Autodesk Fusion 360 part; units mm, degrees
(part 2 of 4)
  spline S0 degree 5 poles (47.3702, 73.019) (47.3923, 73.0171) (47.4364, 73.0131) (47.5026, 73.0067) (47.5909, 72.9976) (47.701, 72.9852) (47.8111, 72.9719) (47.9211, 72.9579) (48.0309, 72.9431) (48.1407, 72.9277) (48.2504, 72.9116) (48.3599, 72.8948) (48.4693, 72.8773) (48.5786, 72.8591) (48.6878, 72.8403) (48.7969, 72.821) (48.9059, 72.8012) (49.0149, 72.7809) (49.1238, 72.7601) (49.2325, 72.7384) (49.341, 72.7156) (49.4491, 72.6914) (49.5568, 72.6656) (49.6641, 72.6381) (49.771, 72.6091) (49.8776, 72.579) (49.984, 72.5482) (50.0903, 72.517) (50.1965, 72.4856) (50.3027, 72.4541) (50.4087, 72.4222) (50.5146, 72.3898) (50.6202, 72.3565) (50.7255, 72.322) (50.8304, 72.2863) (50.9348, 72.2494) (51.0388, 72.2111) (51.1423, 72.1717) (51.2453, 72.1314) (51.3481, 72.0902) (51.4506, 72.0484) (51.5529, 72.0061) (51.6551, 71.9634) (51.7572, 71.9202) (51.859, 71.8765) (51.9604, 71.8319) (52.0614, 71.7862) (52.1617, 71.7392) (52.2614, 71.6908) (52.3603, 71.6411) (52.4587, 71.5903) (52.5566, 71.5385) (52.6542, 71.486) (52.7515, 71.433) (52.8486, 71.3796) (52.9454, 71.3257) (53.0418, 71.2712) (53.1379, 71.2161) (53.2336, 71.1602) (53.3288, 71.1036) (53.4236, 71.0462) (53.5179, 70.9881) (53.6118, 70.9293) (53.7052, 70.8698) (53.7983, 70.8096) (53.8909, 70.7488) (53.983, 70.6873) (54.0746, 70.625) (54.1658, 70.562) (54.2565, 70.4984) (54.3468, 70.4342) (54.4367, 70.3694) (54.5263, 70.3041) (54.6154, 70.2382) (54.704, 70.1716) (54.792, 70.1041) (54.8791, 70.0356) (54.9653, 69.9659) (55.0505, 69.8951) (55.1349, 69.8232) (55.2187, 69.7506) (55.302, 69.6773) (55.3849, 69.6038) (55.4677, 69.53) (55.5503, 69.456) (55.6325, 69.3816) (55.7141, 69.3067) (55.7951, 69.2309) (55.8751, 69.1542) (55.9542, 69.0764) (56.0322, 68.9977) (56.1093, 68.9179) (56.1854, 68.8373) (56.2607, 68.7559) (56.3353, 68.6739) (56.4094, 68.5914) (56.483, 68.5085) (56.5562, 68.4253) (56.6292, 68.3418) (56.7017, 68.2579) (56.7736, 68.1735) (56.8448, 68.0886) (56.9151, 68.0029) (56.9845, 67.9165) (57.053, 67.8293) (57.1207, 67.7416) (57.1877, 67.6533) (57.2542, 67.5646) (57.3203, 67.4756) (57.3859, 67.3862) (57.4509, 67.2965) (57.5153, 67.2063) (57.5788, 67.1155) (57.6414, 67.0241) (57.703, 66.932) (57.7635, 66.8393) (57.8231, 66.7458) (57.8817, 66.6518) (57.9395, 66.5572) (57.9967, 66.4623) (58.0535, 66.3671) (58.11, 66.2718) (58.1661, 66.1765) (58.2219, 66.0809) (58.2771, 65.985) (58.3312, 65.8884) (58.384, 65.791) (58.4353, 65.6925) (58.4851, 65.5931) (58.534, 65.4932) (58.5826, 65.3934) (58.6315, 65.2941) (58.681, 65.1955) (58.7306, 65.0975) (58.7792, 64.9989) (58.8253, 64.8988) (58.8676, 64.796) (58.9055, 64.69) (58.9398, 64.5816) (58.9733, 64.4726) (59.0098, 64.366) (59.0533, 64.2649) (59.1074, 64.1722) (59.1741, 64.0899) (59.2531, 64.0181) (59.3425, 63.956) (59.4393, 63.9018) (59.5404, 63.8534) (59.6431, 63.8089) (59.7459, 63.7665) (59.8483, 63.725) (59.95, 63.6834) (60.0514, 63.6412) (60.1527, 63.598) (60.254, 63.5536) (60.3552, 63.508) (60.4562, 63.4613) (60.5568, 63.4137) (60.6567, 63.3653) (60.7561, 63.316) (60.8548, 63.2659) (60.953, 63.2149) (61.0506, 63.1629) (61.1478, 63.1099) (61.2445, 63.0559) (61.3408, 63.001) (61.4366, 62.9453) (61.532, 62.8889) (61.6269, 62.8317) (61.7214, 62.774) (61.8156, 62.7156) (61.9093, 62.6567) (62.0027, 62.5971) (62.0956, 62.5368) (62.1881, 62.4757) (62.2798, 62.4136) (62.3709, 62.3504) (62.4612, 62.2861) (62.5507, 62.2208) (62.6395, 62.1546) (62.7279, 62.0876) (62.8159, 62.0203) (62.9037, 61.9526) (62.9913, 61.8846) (63.0786, 61.8162) (63.1655, 61.7473) (63.2516, 61.6776) (63.3369, 61.6068) (63.4214, 61.535) (63.505, 61.4623) (63.5881, 61.3889) (63.6708, 61.315) (63.7533, 61.2408) (63.8356, 61.1665) (63.9177, 61.092) (63.9993, 61.017) (64.0804, 60.9414) (64.1606, 60.8649) (64.2398, 60.7874) (64.3181, 60.7088) (64.3954, 60.6293) (64.4718, 60.549) (64.5475, 60.4679) (64.6226, 60.3863) (64.6971, 60.3042) (64.7711, 60.2216) (64.8444, 60.1385) (64.9171, 60.0548) (64.9892, 59.9706) (65.0605, 59.8857) (65.131, 59.8001) (65.2006, 59.7139) (65.2695, 59.627) (65.3375, 59.5396) (65.4049, 59.4515) (65.4716, 59.3631) (65.538, 59.2743) (65.604, 59.1852) (65.6696, 59.0959) (65.7347, 59.0062) (65.7991, 58.916) (65.8628, 58.8254) (65.9255, 58.734) (65.9872, 58.642) (66.0479, 58.5493) (66.1078, 58.4561) (66.167, 58.3624) (66.2255, 58.2683) (66.2835, 58.1739) (66.341, 58.0791) (66.3976, 57.984) (66.4535, 57.8883) (66.5083, 57.7921) (66.5621, 57.6952) (66.615, 57.5979) (66.6671, 57.5001) (66.7186, 57.402) (66.7696, 57.3037) (66.8201, 57.2051) (66.8701, 57.1063) (66.9193, 57.0072) (66.9676, 56.9075) (67.0146, 56.8073) (67.0605, 56.7065) (67.105, 56.6051) (67.1485, 56.5031) (67.191, 56.4008) (67.2327, 56.2981) (67.2736, 56.1951) (67.3138, 56.0919) (67.3531, 55.9884) (67.3915, 55.8846) (67.4289, 55.7804) (67.4654, 55.6759) (67.5012, 55.5711) (67.5367, 55.4662) (67.5721, 55.3612) (67.6075, 55.2562) (67.6429, 55.1511) (67.6779, 55.046) (67.7119, 54.9406) (67.7446, 54.8348) (67.7753, 54.7284) (67.804, 54.6215) (67.831, 54.514) (67.8566, 54.4062) (67.8816, 54.2982) (67.9062, 54.1901) (67.931, 54.0821) (67.9557, 53.9741) (67.98, 53.866) (68.0036, 53.7578) (68.026, 53.6493) (68.0468, 53.5404) (68.0657, 53.4312) (68.0829, 53.3217) (68.0985, 53.2119) (68.1127, 53.1019) (68.1259, 52.9918) (68.1386, 52.8817) (68.1511, 52.7716) (68.1639, 52.6616) (68.1771, 52.5515) (68.1905, 52.4414) (68.2037, 52.3314) (68.2162, 52.2212) (68.2271, 52.1109) (68.2359, 52.0004) (68.2423, 51.8898) (68.2464, 51.779) (68.2486, 51.6681) (68.2492, 51.5571) (68.2491, 51.4462) (68.2487, 51.3353) (68.2484, 51.2244) (68.2484, 51.1135) (68.249, 51.0027) (68.25, 50.8919) (68.2512, 50.781) (68.2522, 50.6701) (68.2526, 50.5592) (68.252, 50.4483) (68.2499, 50.3375) (68.246, 50.2267) (68.2402, 50.116) (68.2327, 50.0054) (68.2235, 49.8949) (68.2129, 49.7846) (68.201, 49.6743) (68.188, 49.5642) (68.1741, 49.4542) (68.1593, 49.3444) (68.1437, 49.2346) (68.1273, 49.125) (68.1105, 49.0155) (68.0932, 48.9061) (68.0755, 48.7966) (68.0574, 48.6872) (68.0388, 48.5779) (68.0194, 48.4687) (67.9988, 48.3598) (67.9766, 48.2512) (67.9528, 48.1431) (67.9273, 48.0353) (67.9003, 47.9279) (67.8725, 47.8207) (67.8444, 47.7135) (67.8164, 47.6063) (67.7886, 47.4991) (67.761, 47.3918) (67.733, 47.2846) (67.7041, 47.1776) (67.6738, 47.0711) (67.6419, 46.9651) (67.6082, 46.8596) (67.5731, 46.7545) (67.5368, 46.6498) (67.4996, 46.5453) (67.4619, 46.4411) (67.4236, 46.3371) (67.3845, 46.2335) (67.3445, 46.1303) (67.3033, 46.0276) (67.2608, 45.9254) (67.2172, 45.8236) (67.1727, 45.7223) (67.1275, 45.6211) (67.0818, 45.5202) (67.0358, 45.4193) (66.9895, 45.3187) (66.9425, 45.2183) (66.8949, 45.1183) (66.8462, 45.0189) (66.7964, 44.92) (66.7453, 44.8217) (66.693, 44.7241) (66.6397, 44.6269) (66.5853, 44.5303) (66.5302, 44.434) (66.4745, 44.3381) (66.4185, 44.2425) (66.3621, 44.1472) (66.3054, 44.0523) (66.2481, 43.9579) (66.1898, 43.8641) (66.1299, 43.771) (66.068, 43.6788) (66.0041, 43.5874) (65.9387, 43.4968) (65.8727, 43.4066) (65.8076, 43.3164) (65.7444, 43.226) (65.6835, 43.1351) (65.6241, 43.0442) (65.5635, 42.9539) (65.4987, 42.8653) (65.4271, 42.779) (65.3476, 42.6953) (65.262, 42.6138) (65.1757, 42.5327) (65.0966, 42.4495) (65.0324, 42.3619) (64.9895, 42.268) (64.9708, 42.1668) (64.9739, 42.0591) (64.993, 41.9468) (65.0204, 41.8321) (65.0488, 41.7174) (65.0725, 41.6043) (65.0895, 41.4934) (65.1006, 41.3843) (65.108, 41.2762) (65.1145, 41.1681) (65.1223, 41.0592) (65.132, 40.9494) (65.143, 40.8386) (65.1542, 40.7272) (65.1642, 40.6157) (65.1719, 40.5044) (65.177, 40.3934) (65.1797, 40.2827) (65.1808, 40.1722) (65.1809, 40.0617) (65.1806, 39.9511) (65.1803, 39.8403) (65.1799, 39.7294) (65.1793, 39.6184) (65.1784, 39.5073) (65.1767, 39.3964) (65.1741, 39.2855) (65.1703, 39.1747) (65.1654, 39.064) (65.1591, 38.9534) (65.1516, 38.8428) (65.1429, 38.7322) (65.1332, 38.6218) (65.1226, 38.5114) (65.1114, 38.4011) (65.0995, 38.2908) (65.0871, 38.1807) (65.0742, 38.0707) (65.0605, 37.9607) (65.0461, 37.8509) (65.0307, 37.7411) (65.0142, 37.6315) (64.9965, 37.5221) (64.9775, 37.4129) (64.9571, 37.304) (64.9355, 37.1954) (64.9127, 37.087) (64.889, 36.9787) (64.8648, 36.8706) (64.8401, 36.7626) (64.8151, 36.6547) (64.7896, 36.5468) (64.7633, 36.4392) (64.736, 36.3319) (64.7073, 36.2249) (64.6772, 36.1183) (64.6457, 36.0121) (64.6128, 35.9063) (64.579, 35.8008) (64.5443, 35.6956) (64.5091, 35.5905) (64.4735, 35.4857) (64.4373, 35.381) (64.4007, 35.2765) (64.3635, 35.1722) (64.3256, 35.0681) (64.287, 34.9643) (64.2476, 34.8608) (64.2074, 34.7576) (64.1664, 34.6547) (64.1246, 34.5521) (64.082, 34.4499) (64.0386, 34.348) (63.9944, 34.2465) (63.9493, 34.1453) (63.9035, 34.0444) (63.857, 33.9439) (63.8099, 33.8435) (63.7623, 33.7435) (63.7141, 33.6436) (63.6655, 33.544) (63.6161, 33.4448) (63.5659, 33.346) (63.5147, 33.2478) (63.4623, 33.1502) (63.4087, 33.0533) (63.3539, 32.957) (63.2981, 32.8613) (63.2414, 32.7661) (63.184, 32.6713) (63.126, 32.5769) (63.0673, 32.4828) (63.0079, 32.3893) (62.9475, 32.2963) (62.8862, 32.204) (62.8238, 32.1124) (62.7604, 32.0215) (62.6962, 31.9312) (62.6312, 31.8414) (62.5657, 31.752) (62.4997, 31.6629) (62.4333, 31.5741) (62.3665, 31.4857) (62.2992, 31.3977) (62.2313, 31.3101) (62.1627, 31.2231) (62.0935, 31.1365) (62.0235, 31.0505) (61.953, 30.9651) (61.8817, 30.8801) (61.8098, 30.7958) (61.7372, 30.712) (61.6638, 30.6289) (61.5896, 30.5464) (61.5146, 30.4648) (61.4388, 30.3839) (61.3621, 30.3038) (61.2847, 30.2244) (61.2065, 30.1458) (61.1277, 30.0678) (61.0483, 29.9904) (60.9684, 29.9136) (60.8879, 29.8374) (60.8069, 29.7617) (60.7253, 29.6866) (60.6431, 29.6121) (60.5603, 29.5384) (60.4769, 29.4653) (60.3928, 29.3931) (60.308, 29.3217) (60.2225, 29.2511) (60.1365, 29.1812) (60.05, 29.1119) (59.9631, 29.0431) (59.876, 28.9746) (59.7885, 28.9064) (59.7007, 28.8388) (59.6124, 28.7719) (59.5234, 28.7058) (59.4336, 28.6409) (59.3429, 28.5772) (59.2515, 28.5146) (59.1594, 28.4529) (59.0668, 28.392) (58.9739, 28.3315) (58.8807, 28.2715) (58.7873, 28.2119) (58.6936, 28.1529) (58.5994, 28.0945) (58.5047, 28.0371) (58.4095, 27.9806) (58.3137, 27.925) (58.2174, 27.8702) (58.1209, 27.8159) (58.024, 27.7621) (57.927, 27.7087) (57.8297, 27.6558) (57.732, 27.6037) (57.6338, 27.5527) (57.535, 27.503) (57.4355, 27.4546) (57.3353, 27.4076) (57.2346, 27.3616) (57.1334, 27.3166) (57.032, 27.2721) (56.9303, 27.2282) (56.8285, 27.1847) (56.7264, 27.1418) (56.624, 27.0997) (56.5212, 27.0585) (56.418, 27.0183) (56.3144, 26.9791) (56.2105, 26.9407) (56.1063, 26.903) (56.0018, 26.8659) (55.8971, 26.8295) (55.7922, 26.7937) (55.687, 26.7591) (55.5814, 26.7257) (55.4753, 26.6939) (55.3689, 26.6635) (55.262, 26.6345) (55.1549, 26.6063) (55.0476, 26.5787) (54.9402, 26.5511) (54.8329, 26.5235) (54.7256, 26.4959) (54.6181, 26.4688) (54.5105, 26.4426) (54.4026, 26.4177) (54.2944, 26.3943) (54.1858, 26.3723) (54.077, 26.3513) (53.968, 26.3311) (53.8588, 26.3113) (53.7496, 26.2919) (53.6403, 26.273) (53.5309, 26.2551) (53.4213, 26.2387) (53.3115, 26.2242) (53.2014, 26.2116) (53.0911, 26.2007) (52.9807, 26.1907) (52.8702, 26.181) (52.7597, 26.171) (52.6493, 26.1604) (52.539, 26.1494) (52.4286, 26.1387) (52.3183, 26.1288) (52.2078, 26.1205) (52.0972, 26.1142) (51.9865, 26.1101) (51.8756, 26.1079) (51.7647, 26.1071) (51.6536, 26.1072) (51.5426, 26.1078) (51.4317, 26.1084) (51.3208, 26.109) (51.21, 26.1096) (51.0993, 26.1102) (50.9886, 26.1112) (50.8779, 26.1129) (50.7672, 26.1159) (50.6563, 26.1205) (50.5453, 26.1271) (50.4342, 26.1356) (50.3233, 26.1459) (50.2128, 26.1574) (50.1028, 26.1697) (49.9935, 26.1823) (49.8846, 26.195) (49.7756, 26.208) (49.6661, 26.2213) (49.5555, 26.235) (49.4438, 26.2481) (49.3315, 26.2586) (49.2199, 26.2633) (49.1109, 26.2578) (49.0064, 26.2384) (48.9077, 26.2025) (48.8154, 26.1498) (48.7284, 26.0829) (48.6448, 26.0066) (48.5626, 25.9264) (48.4795, 25.8474) (48.3941, 25.7732) (48.3062, 25.7048) (48.216, 25.6412) (48.1244, 25.5805) (48.0325, 25.5205) (47.9409, 25.4593) (47.8498, 25.3965) (47.759, 25.3327) (47.6681, 25.2686) (47.5766, 25.2053) (47.4842, 25.1438) (47.3907, 25.084) (47.2965, 25.0259) (47.2016, 24.9689) (47.1065, 24.9124) (47.0112, 24.8561) (46.9157, 24.8) (46.82, 24.7442) (46.724, 24.6891) (46.6273, 24.6349) (46.5299, 24.5821) (46.4318, 24.5306) (46.333, 24.4803) (46.2336, 24.4312) (46.1339, 24.383) (46.0337, 24.3356) (45.9333, 24.2889) (45.8326, 24.2429) (45.7316, 24.1976) (45.6302, 24.153) (45.5286, 24.1092) (45.4266, 24.0661) (45.3242, 24.0238) (45.2215, 23.9823) (45.1186, 23.9415) (45.0152, 23.9015) (44.9115, 23.8626) (44.8074, 23.8248) (44.7029, 23.7883) (44.5979, 23.753) (44.4926, 23.719) (44.3869, 23.686) (44.281, 23.6537) (44.1749, 23.6217) (44.0688, 23.5899) (43.9626, 23.5582) (43.8564, 23.5269) (43.7499, 23.4963) (43.6431, 23.4671) (43.5358, 23.4394) (43.4281, 23.4137) (43.32, 23.3897) (43.2115, 23.3672) (43.1027, 23.3459) (42.9937, 23.3252) (42.8848, 23.3051) (42.7757, 23.2853) (42.6666, 23.266) (42.5575, 23.2473) (42.4482, 23.2292) (42.3388, 23.212) (42.2292, 23.1955) (42.1195, 23.1795) (42.0097, 23.1641) (41.8999, 23.149) (41.7899, 23.1344) (41.6799, 23.1204) (41.5699, 23.1073) (41.4596, 23.0954) (41.3493, 23.085) (41.2388, 23.0763) (41.1282, 23.0693) (41.0174, 23.0639) (40.9066, 23.06) (40.7957, 23.0572) (40.6848, 23.0554) (40.5739, 23.0543) (40.463, 23.0538) (40.3522, 23.0535) (40.2414, 23.0535) (40.1305, 23.0537) (40.0197, 23.0539) (39.9088, 23.0544) (39.7979, 23.055) (39.687, 23.0561) (39.5761, 23.0579) (39.4652, 23.0608) (39.3544, 23.0651) (39.2437, 23.0712) (39.1332, 23.0794) (39.0228, 23.0897) (38.9127, 23.1019) (38.8026, 23.1154) (38.6927, 23.1299) (38.5828, 23.1449) (38.4729, 23.1601) (38.3631, 23.1755) (38.2534, 23.1913) (38.1439, 23.2076) (38.0344, 23.2247) (37.9251, 23.2426) (37.816, 23.2614) (37.7069, 23.2808) (37.5979, 23.3006) (37.4889, 23.3207) (37.3799, 23.3412) (37.271, 23.3623) (37.1624, 23.3844) (37.0542, 23.408) (36.9464, 23.4333) (36.8391, 23.4605) (36.7321, 23.4893) (36.6255, 23.5192) (36.5189, 23.5497) (36.4124, 23.5801) (36.3057, 23.6104) (36.1991, 23.6405) (36.0926, 23.671) (35.9863, 23.7022) (35.8805, 23.7347) (35.7751, 23.7689) (35.6704, 23.8048) (35.5661, 23.8422) (35.4624, 23.881) (35.359, 23.9208) (35.2559, 23.9614) (35.1531, 24.0025) (35.0504, 24.0441) (34.948, 24.0861) (34.8457, 24.1285) (34.7436, 24.1716) (34.6419, 24.2155) (34.5407, 24.2605) (34.4401, 24.3067) (34.3402, 24.3544) (34.241, 24.4034) (34.1424, 24.4536) (34.0442, 24.5048) (33.9463, 24.5565) (33.8486, 24.6084) (33.7508, 24.6605) (33.6532, 24.7128) (33.5558, 24.7654) (33.4586, 24.8187) (33.362, 24.8728) (33.266, 24.9281) (33.1706, 24.9844) (33.0759, 25.0419) (32.9818, 25.1004) (32.8882, 25.1598) (32.7951, 25.2199) (32.7024, 25.2806) (32.61, 25.3418) (32.5179, 25.4034) (32.426, 25.4654) (32.3345, 25.5278) (32.2432, 25.5907) (32.1524, 25.6542) (32.062, 25.7183) (31.9723, 25.7834) (31.8832, 25.8493) (31.7947, 25.9161) (31.707, 25.9839) (31.6199, 26.0525) (31.5336, 26.122) (31.4478, 26.1923) (31.3627, 26.2634) (31.2782, 26.3352) (31.1943, 26.4077) (31.111, 26.4809) (31.0283, 26.5547) (30.9462, 26.6291) (30.8647, 26.7042) (30.7837, 26.78) (30.7033, 26.8563) (30.6235, 26.9333) (30.5444, 27.011) (30.466, 27.0895) (30.3884, 27.1686) (30.3116, 27.2486) (30.2356, 27.3293) (30.1603, 27.4106) (30.0856, 27.4926) (30.0116, 27.5751) (29.9381, 27.6581) (29.865, 27.7415) (29.7925, 27.8253) (29.7204, 27.9096) (29.649, 27.9944) (29.5783, 28.0798) (29.5084, 28.1659) (29.4393, 28.2526) (29.3711, 28.34) (29.3038, 28.4281) (29.2374, 28.5168) (29.1717, 28.6061) (29.1069, 28.696) (29.0426, 28.7863) (28.979, 28.877) (28.9158, 28.968) (28.8531, 29.0594) (28.7909, 29.1511) (28.7293, 29.2432) (28.6685, 29.3359) (28.6086, 29.4291) (28.5496, 29.523) (28.4916, 29.6174) (28.4345, 29.7124) (28.3783, 29.8078) (28.3229, 29.9037) (28.2684, 30.0001) (28.2146, 30.0969) (28.1617, 30.1942) (28.1097, 30.292) (28.0585, 30.3904) (28.0079, 30.4891) (27.9577, 30.5881) (27.9076, 30.6869) (27.8573, 30.7853) (27.807, 30.8835) (27.7572, 30.9817) (27.7089, 31.0807) (27.6633, 31.1813) (27.6214, 31.2842) (27.5834, 31.3899) (27.5486, 31.4975) (27.5144, 31.6056) (27.4775, 31.7117) (27.4343, 31.813) (27.3816, 31.9073) (27.3175, 31.9925) (27.242, 32.0681) (27.1564, 32.1342) (27.0629, 32.1917) (26.9642, 32.2423) (26.8626, 32.2876) (26.7596, 32.3295) (26.6565, 32.3698) (26.5537, 32.4102) (26.4516, 32.4519) (26.3502, 32.4956) (26.2494, 32.5415) (26.1492, 32.5891) (26.0495, 32.6379) (25.95, 32.6872) (25.8507, 32.7367) (25.7517, 32.7864) (25.6529, 32.8363) (25.5545, 32.8867) (25.4565, 32.9381) (25.3591, 32.9907) (25.2622, 33.0444) (25.1658, 33.0991) (25.0698, 33.1547) (24.9743, 33.211) (24.8791, 33.2677) (24.7842, 33.3249) (24.6896, 33.3824) (24.5953, 33.4405) (24.5013, 33.4991) (24.4078, 33.5585) (24.3148, 33.6187) (24.2224, 33.68) (24.1309, 33.7426) (24.0402, 33.8063) (23.9504, 33.8713) (23.8614, 33.9373) (23.773, 34.0041) (23.685, 34.0715) (23.5973, 34.1394) (23.51, 34.2076) (23.4229, 34.2762) (23.3362, 34.3454) (23.2502, 34.4153) (23.1648, 34.486) (23.0802, 34.5576) (22.9964, 34.6302) (22.9132, 34.7035) (22.8305, 34.7774) (22.7482, 34.8517) (22.6663, 34.9264) (22.5847, 35.0014) (22.5034, 35.0768) (22.4226, 35.1527) (22.3424, 35.2293) (22.2629, 35.3065) (22.1841, 35.3846) (22.1063, 35.4636) (22.0295, 35.5436) (21.9536, 35.6244) (21.8787, 35.7061) (21.8046, 35.7885) (21.731, 35.8715) (21.6579, 35.9548) (21.5851, 36.0385) (21.5126, 36.1224) (21.4406, 36.2067) (21.3692, 36.2915) (21.2988, 36.3771) (21.2295, 36.4635) (21.1613, 36.5509) (21.0942, 36.639) (21.0278, 36.7278) (20.9618, 36.8169) (20.8962, 36.9062) (20.8306, 36.9956) (20.7654, 37.0852) (20.7007, 37.1753) (20.6369, 37.2659) (20.5742, 37.3572) (20.5129, 37.4495) (20.4527, 37.5426) (20.3936, 37.6364) (20.3352, 37.7306) (20.2774, 37.8252) (20.2199, 37.9199) (20.1627, 38.0148) (20.1059, 38.1099) (20.0495, 38.2052) (19.9937, 38.3009) (19.9387, 38.397) (19.8845, 38.4936) (19.8313, 38.5907) (19.779, 38.6883) (19.7278, 38.7865) (19.6775, 38.8851) (19.6282, 38.9841) (19.5798, 39.0837) (19.5324, 39.1837) (19.4859, 39.2842) (19.4403, 39.3851) (19.3956, 39.4865) (19.3519, 39.5883) (19.3091, 39.6905) (19.2674, 39.7931) (19.2267, 39.8961) (19.187, 39.9995) (19.1482, 40.1032) (19.1103, 40.2072) (19.0731, 40.3115) (19.0365, 40.416) (19.0004, 40.5207) (18.9645, 40.6256) (18.9289, 40.7305) (18.8935, 40.8355) (18.8585, 40.9407) (18.8242, 41.0461) (18.7911, 41.1518) (18.7596, 41.258) (18.73, 41.3647) (18.7024, 41.4719) (18.6766, 41.5797) (18.6522, 41.6878) (18.6288, 41.7961) (18.6059, 41.9046) (18.5831, 42.0131) (18.5604, 42.1215) (18.5378, 42.23) (18.5156, 42.3385) (18.494, 42.4471) (18.4732, 42.556) (18.4534, 42.665) (18.4347, 42.7742) (18.4172, 42.8836) (18.4007, 42.9932) (18.3852, 43.1029) (18.3703, 43.2127) (18.3558, 43.3225) (18.3412, 43.4324) (18.3267, 43.5423) (18.3122, 43.6523) (18.2983, 43.7623) (18.2854, 43.8724) (18.2743, 43.9827) (18.2655, 44.0932) (18.2591, 44.2038) (18.2551, 44.3146) (18.253, 44.4255) (18.2522, 44.5364) (18.2522, 44.6474) (18.2523, 44.7583) (18.2523, 44.8691) (18.2519, 44.9799) (18.2513, 45.0908) (18.2506, 45.2017) (18.2502, 45.3126) (18.2506, 45.4236) (18.2525, 45.5345) (18.2563, 45.6453) (18.2626, 45.7559) (18.2712, 45.8664) (18.2818, 45.9767) (18.2939, 46.0869) (18.3067, 46.1971) (18.3195, 46.3072) (18.3321, 46.4174) (18.3443, 46.5275) (18.3564, 46.6377) (18.3687, 46.7478) (18.3818, 46.8579) (18.3959, 46.9678) (18.4114, 47.0776) (18.4283, 47.1872) (18.4466, 47.2965) (18.4663, 47.4056) (18.4871, 47.5145) (18.5089, 47.6231) (18.5315, 47.7316) (18.5546, 47.8399) (18.5783, 47.9482) (18.6024, 48.0564) (18.6272, 48.1644) (18.6528, 48.2721) (18.6795, 48.3796) (18.7075, 48.4868) (18.7367, 48.5936) (18.7672, 48.7001) (18.7986, 48.8063) (18.8307, 48.9123) (18.8633, 49.0181) (18.8963, 49.1239) (18.9297, 49.2294) (18.9638, 49.3348) (18.9988, 49.4399) (19.0349, 49.5445) (19.0722, 49.6488) (19.1107, 49.7526) (19.1504, 49.856) (19.1909, 49.9591) (19.2322, 50.0618) (19.2739, 50.1644) (19.316, 50.2667) (19.3585, 50.369) (19.4013, 50.4711) (19.4445, 50.5731) (19.4884, 50.6749) (19.533, 50.7764) (19.5786, 50.8774) (19.6255, 50.9778) (19.6738, 51.0775) (19.7236, 51.1764) (19.7748, 51.2746) (19.8274, 51.3722) (19.881, 51.4692) (19.9354, 51.5659) (19.9905, 51.6622) (20.0458, 51.7583) (20.1013, 51.8542) (20.1569, 51.95) (20.2126, 52.0454) (20.2687, 52.1405) (20.3257, 52.235) (20.3842, 52.329) (20.4445, 52.4222) (20.5068, 52.5147) (20.5706, 52.6066) (20.6348, 52.6981) (20.698, 52.7895) (20.7593, 52.8812) (20.8183, 52.9731) (20.8759, 53.0649) (20.9349, 53.156) (20.9985, 53.2454) (21.0694, 53.3325) (21.1485, 53.4172) (21.2339, 53.4999) (21.3196, 53.5824) (21.3975, 53.6668) (21.4593, 53.7555) (21.4987, 53.8501) (21.5128, 53.9516) (21.5047, 54.0592) (21.481, 54.1713) (21.4501, 54.2857) (21.4201, 54.4002) (21.3968, 54.5133) (21.3817, 54.6244) (21.3735, 54.734) (21.3691, 54.8425) (21.365, 54.9509) (21.3585, 55.06) (21.349, 55.1699) (21.3374, 55.2806) (21.3254, 55.3918) (21.315, 55.5032) (21.3075, 55.6144) (21.3033, 55.7254) (21.302, 55.8362) (21.3026, 55.9468) (21.3041, 56.0573) (21.3055, 56.168) (21.3063, 56.2788) (21.3064, 56.3897) (21.3061, 56.5006) (21.3056, 56.6117) (21.3055, 56.7227) (21.3064, 56.8337) (21.3088, 56.9445) (21.313, 57.0553) (21.3193, 57.1659) (21.3277, 57.2763) (21.3377, 57.3867) (21.3488, 57.497) (21.3604, 57.6073) (21.3718, 57.7176) (21.3828, 57.828) (21.3936, 57.9383) (21.4045, 58.0486) (21.416, 58.1588) (21.4287, 58.269) (21.443, 58.3789) (21.4593, 58.4886) (21.4776, 58.5979) (21.4978, 58.707) (21.5196, 58.8157) (21.5428, 58.924) (21.567, 59.0321) (21.5918, 59.1401) (21.6169, 59.248) (21.6422, 59.3559) (21.6675, 59.4637) (21.6933, 59.5715) (21.7199, 59.6791) (21.7476, 59.7864) (21.7768, 59.8932) (21.8077, 59.9996) (21.8402, 60.1054) (21.8739, 60.211) (21.9084, 60.3162) (21.9434, 60.4214) (21.9786, 60.5264) (22.014, 60.6314) (22.0497, 60.7362) (22.086, 60.8408) (22.1231, 60.9451) (22.1611, 61.0491) (22.2001, 61.1527) (22.2398, 61.2561) (22.2801, 61.3593) (22.3208, 61.4624) (22.362, 61.5652) (22.4037, 61.6679) (22.4461, 61.7702) (22.4896, 61.8721) (22.5344, 61.9733) (22.5804, 62.074) (22.6276, 62.1741) (22.6757, 62.2739) (22.7243, 62.3733) (22.7732, 62.4727) (22.8223, 62.5719) (22.8717, 62.671) (22.9216, 62.7697) (22.9726, 62.868) (23.0247, 62.9656) (23.0783, 63.0625) (23.1333, 63.1586) (23.1894, 63.2542) (23.2464, 63.3493) (23.3041, 63.4439) (23.3623, 63.5383) (23.4211, 63.6322) (23.4805, 63.7257) (23.5408, 63.8186) (23.6021, 63.9109) (23.6645, 64.0024) (23.7279, 64.0932) (23.7922, 64.1835) (23.8571, 64.2734) (23.9225, 64.363) (23.9881, 64.4523) (24.0541, 64.5414) (24.1206, 64.6301) (24.1877, 64.7183) (24.2555, 64.8058) (24.3243, 64.8927) (24.3939, 64.9789) (24.4643, 65.0646) (24.5353, 65.1497) (24.6068, 65.2345) (24.6787, 65.3189) (24.7512, 65.4028) (24.8242, 65.4862) (24.898, 65.5689) (24.9727, 65.6508) (25.0484, 65.7318) (25.1249, 65.8121) (25.2021, 65.8916) (25.28, 65.9705) (25.3584, 66.049) (25.4371, 66.1271) (25.5163, 66.2048) (25.596, 66.2818) (25.6764, 66.3581) (25.7577, 66.4335) (25.8399, 66.5079) (25.9232, 66.5811) (26.0074, 66.6533) (26.0924, 66.7244) (26.1783, 66.7945) (26.2647, 66.8639) (26.3517, 66.9326) (26.439, 67.0008) (26.5265, 67.0688) (26.6141, 67.1367) (26.7019, 67.2043) (26.79, 67.2716) (26.8785, 67.3384) (26.9675, 67.4044) (27.0573, 67.4693) (27.1478, 67.5332) (27.2391, 67.596) (27.331, 67.6579) (27.4233, 67.7191) (27.516, 67.7799) (27.609, 67.8401) (27.7024, 67.8999) (27.7961, 67.959) (27.8903, 68.0172) (27.9852, 68.0743) (28.0806, 68.1304) (28.1767, 68.1855) (28.2732, 68.2398) (28.37, 68.2937) (28.4669, 68.3474) (28.5639, 68.4008) (28.6612, 68.4538) (28.7588, 68.5061) (28.8569, 68.5572) (28.9558, 68.6069) (29.0554, 68.6551) (29.1557, 68.7017) (29.2566, 68.7472) (29.358, 68.7918) (29.4596, 68.836) (29.5613, 68.8799) (29.6631, 68.9234) (29.7651, 68.9665) (29.8674, 69.0089) (29.9701, 69.0502) (30.0732, 69.0905) (30.1769, 69.1296) (30.2809, 69.1678) (30.3852, 69.2052) (30.4898, 69.242) (30.5945, 69.2782) (30.6995, 69.3137) (30.8048, 69.3482) (30.9104, 69.3815) (31.0165, 69.4133) (31.123, 69.4436) (31.2299, 69.4727) (31.337, 69.5008) (31.4444, 69.5283) (31.5517, 69.5557) (31.6591, 69.5831) (31.7665, 69.6103) (31.874, 69.6371) (31.9816, 69.6632) (32.0895, 69.688) (32.1977, 69.7116) (32.3063, 69.7338) (32.4151, 69.7549) (32.5241, 69.7752) (32.6332, 69.7949) (32.7425, 69.814) (32.8519, 69.8323) (32.9614, 69.8495) (33.0711, 69.8652) (33.181, 69.8791) (33.2912, 69.8912) (33.4015, 69.902) (33.5119, 69.912) (33.6223, 69.9218) (33.7328, 69.9322) (33.8432, 69.9432) (33.9535, 69.9545) (34.0638, 69.9657) (34.1742, 69.9758) (34.2846, 69.9843) (34.3952, 69.9906) (34.5059, 69.9947) (34.6168, 69.997) (34.7277, 69.998) (34.8387, 69.9982) (34.9498, 69.9981) (35.0607, 69.9978) (35.1716, 69.9975) (35.2824, 69.9969) (35.3931, 69.9958) (35.5038, 69.9939) (35.6144, 69.9911) (35.7251, 69.9872) (35.836, 69.9819) (35.947, 69.9752) (36.058, 69.9671) (36.169, 69.9575) (36.2795, 69.9467) (36.3896, 69.9346) (36.4989, 69.9215) (36.6078, 69.9076) (36.7167, 69.8929) (36.8261, 69.8779) (36.9365, 69.8632) (37.048, 69.8503) (37.1601, 69.8412) (37.2713, 69.8392) (37.3799, 69.8479) (37.4842, 69.8705) (37.5828, 69.9088) (37.6753, 69.9628) (37.7627, 70.0296) (37.8468, 70.1048) (37.9298, 70.1833) (38.0138, 70.2604) (38.1, 70.3328) (38.1889, 70.3998) (38.2799, 70.4623) (38.3721, 70.5223) (38.4647, 70.5818) (38.5568, 70.6425) (38.6483, 70.7047) (38.7395, 70.768) (38.8307, 70.8315) (38.9225, 70.8941) (39.0152, 70.955) (39.1089, 71.0142) (39.2035, 71.0717) (39.2988, 71.1281) (39.3944, 71.1839) (39.4903, 71.2394) (39.5864, 71.2946) (39.6829, 71.3492) (39.7798, 71.4029) (39.8773, 71.4556) (39.9754, 71.5069) (40.0742, 71.5569) (40.1735, 71.606) (40.2731, 71.6543) (40.3729, 71.7023) (40.4729, 71.7499) (40.5731, 71.7972) (40.6735, 71.844) (40.7743, 71.89) (40.8755, 71.935) (40.9773, 71.9788) (41.0796, 72.0213) (41.1823, 72.0625) (41.2855, 72.1027) (41.3891, 72.1419) (41.4929, 72.1803) (41.597, 72.2181) (41.7012, 72.2553) (41.8057, 72.2922) (41.9103, 72.3286) (42.0151, 72.3645) (42.1201, 72.3997) (42.2254, 72.4342) (42.331, 72.4675) (42.437, 72.4998) (42.5433, 72.5307) (42.6499, 72.5606) (42.7569, 72.5895) (42.864, 72.6176) (42.9714, 72.6451) (43.0789, 72.672) (43.1865, 72.6982) (43.2944, 72.7235) (43.4025, 72.7478) (43.5109, 72.7707) (43.6195, 72.7924) (43.7284, 72.8129) (43.8375, 72.8324) (43.9467, 72.8513) (44.0561, 72.8696) (44.1655, 72.8875) (44.275, 72.9049) (44.3846, 72.9215) (44.4943, 72.9372) (44.6042, 72.9516) (44.7142, 72.9649) (44.8244, 72.9771) (44.9346, 72.9884) (45.045, 72.9991) (45.1554, 73.0095) (45.2659, 73.0195) (45.3764, 73.0289) (45.4869, 73.0373) (45.5975, 73.0443) (45.7082, 73.0496) (45.8189, 73.053) (45.9298, 73.0549) (46.0406, 73.0556) (46.1516, 73.0555) (46.2625, 73.0553) (46.3734, 73.055) (46.4843, 73.0546) (46.5952, 73.0541) (46.706, 73.0529) (46.8168, 73.0508) (46.9276, 73.0474) (47.0384, 73.0426) (47.1491, 73.0363) (47.2376, 73.03) (47.3039, 73.0248) (47.3481, 73.021) (47.3702, 73.019) knots 0 0 0 0 0 0 0.0006993 0.0013986 0.0020979 0.0027972 0.0034965 0.0041958 0.0048951 0.00559441 0.00629371 0.00699301 0.00769231 0.00839161 0.00909091 0.00979021 0.01048951 0.01118881 0.01188811 0.01258741 0.01328671 0.01398601 0.01468531 0.01538462 0.01608392 0.01678322 0.01748252 0.01818182 0.01888112 0.01958042 0.02027972 0.02097902 0.02167832 0.02237762 0.02307692 0.02377622 0.02447552 0.02517483 0.02587413 0.02657343 0.02727273 0.02797203 0.02867133 0.02937063 0.03006993 0.03076923 0.03146853 0.03216783 0.03286713 0.03356643 0.03426573 0.03496503 0.03566434 0.03636364 0.03706294 0.03776224 0.03846154 0.03916084 0.03986014 0.04055944 0.04125874 0.04195804 0.04265734 0.04335664 0.04405594 0.04475524 0.04545455 0.04615385 0.04685315 0.04755245 0.04825175 0.04895105 0.04965035 0.05034965 0.05104895 0.05174825 0.05244755 0.05314685 0.05384615 0.05454545 0.05524476 0.05594406 0.05664336 0.05734266 0.05804196 0.05874126 0.05944056 0.06013986 0.06083916 0.06153846 0.06223776 0.06293706 0.06363636 0.06433566 0.06503497 0.06573427 0.06643357 0.06713287 0.06783217 0.06853147 0.06923077 0.06993007 0.07062937 0.07132867 0.07202797 0.07272727 0.07342657 0.07412587 0.07482517 0.07552448 0.07622378 0.07692308 0.07762238 0.07832168 0.07902098 0.07972028 0.08041958 0.08111888 0.08181818 0.08251748 0.08321678 0.08391608 0.08461538 0.08531469 0.08601399 0.08671329 0.08741259 0.08811189 0.08881119 0.08951049 0.09020979 0.09090909 0.09160839 0.09230769 0.09300699 0.09370629 0.09440559 0.0951049 0.0958042 0.0965035 0.0972028 0.0979021 0.0986014 0.0993007 0.1 0.1006993 0.1013986 0.1020979 0.1027972 0.1034965 0.1041958 0.1048951 0.10559441 0.10629371 0.10699301 0.10769231 0.10839161 0.10909091 0.10979021 0.11048951 0.11118881 0.11188811 0.11258741 0.11328671 0.11398601 0.11468531 0.11538462 0.11608392 0.11678322 0.11748252 0.11818182 0.11888112 0.11958042 0.12027972 0.12097902 0.12167832 0.12237762 0.12307692 0.12377622 0.12447552 0.12517483 0.12587413 0.12657343 0.12727273 0.12797203 0.12867133 0.12937063 0.13006993 0.13076923 0.13146853 0.13216783 0.13286713 0.13356643 0.13426573 0.13496503 0.13566434 0.13636364 0.13706294 0.13776224 0.13846154 0.13916084 0.13986014 0.14055944 0.14125874 0.14195804 0.14265734 0.14335664 0.14405594 0.14475524 0.14545455 0.14615385 0.14685315 0.14755245 0.14825175 0.14895105 0.14965035 0.15034965 0.15104895 0.15174825 0.15244755 0.15314685 0.15384615 0.15454545 0.15524476 0.15594406 0.15664336 0.15734266 0.15804196 0.15874126 0.15944056 0.16013986 0.16083916 0.16153846 0.16223776 0.16293706 0.16363636 0.16433566 0.16503497 0.16573427 0.16643357 0.16713287 0.16783217 0.16853147 0.16923077 0.16993007 0.17062937 0.17132867 0.17202797 0.17272727 0.17342657 0.17412587 0.17482517 0.17552448 0.17622378 0.17692308 0.17762238 0.17832168 0.17902098 0.17972028 0.18041958 0.18111888 0.18181818 0.18251748 0.18321678 0.18391608 0.18461538 0.18531469 0.18601399 0.18671329 0.18741259 0.18811189 0.18881119 0.18951049 0.19020979 0.19090909 0.19160839 0.19230769 0.19300699 0.19370629 0.19440559 0.1951049 0.1958042 0.1965035 0.1972028 0.1979021 0.1986014 0.1993007 0.2 0.2006993 0.2013986 0.2020979 0.2027972 0.2034965 0.2041958 0.2048951 0.20559441 0.20629371 0.20699301 0.20769231 0.20839161 0.20909091 0.20979021 0.21048951 0.21118881 0.21188811 0.21258741 0.21328671 0.21398601 0.21468531 0.21538462 0.21608392 0.21678322 0.21748252 0.21818182 0.21888112 0.21958042 0.22027972 0.22097902 0.22167832 0.22237762 0.22307692 0.22377622 0.22447552 0.22517483 0.22587413 0.22657343 0.22727273 0.22797203 0.22867133 0.22937063 0.23006993 0.23076923 0.23146853 0.23216783 0.23286713 0.23356643 0.23426573 0.23496503 0.23566434 0.23636364 0.23706294 0.23776224 0.23846154 0.23916084 0.23986014 0.24055944 0.24125874 0.24195804 0.24265734 0.24335664 0.24405594 0.24475524 0.24545455 0.24615385 0.24685315 0.24755245 0.24825175 0.24895105 0.24965035 0.25034965 0.25104895 0.25174825 0.25244755 0.25314685 0.25384615 0.25454545 0.25524476 0.25594406 0.25664336 0.25734266 0.25804196 0.25874126 0.25944056 0.26013986 0.26083916 0.26153846 0.26223776 0.26293706 0.26363636 0.26433566 0.26503497 0.26573427 0.26643357 0.26713287 0.26783217 0.26853147 0.26923077 0.26993007 0.27062937 0.27132867 0.27202797 0.27272727 0.27342657 0.27412587 0.27482517 0.27552448 0.27622378 0.27692308 0.27762238 0.27832168 0.27902098 0.27972028 0.28041958 0.28111888 0.28181818 0.28251748 0.28321678 0.28391608 0.28461538 0.28531469 0.28601399 0.28671329 0.28741259 0.28811189 0.28881119 0.28951049 0.29020979 0.29090909 0.29160839 0.29230769 0.29300699 0.29370629 0.29440559 0.2951049 0.2958042 0.2965035 0.2972028 0.2979021 0.2986014 0.2993007 0.3 0.3006993 0.3013986 0.3020979 0.3027972 0.3034965 0.3041958 0.3048951 0.30559441 0.30629371 0.30699301 0.30769231 0.30839161 0.30909091 0.30979021 0.31048951 0.31118881 0.31188811 0.31258741 0.31328671 0.31398601 0.31468531 0.31538462 0.31608392 0.31678322 0.31748252 0.31818182 0.31888112 0.31958042 0.32027972 0.32097902 0.32167832 0.32237762 0.32307692 0.32377622 0.32447552 0.32517483 0.32587413 0.32657343 0.32727273 0.32797203 0.32867133 0.32937063 0.33006993 0.33076923 0.33146853 0.33216783 0.33286713 0.33356643 0.33426573 0.33496503 0.33566434 0.33636364 0.33706294 0.33776224 0.33846154 0.33916084 0.33986014 0.34055944 0.34125874 0.34195804 0.34265734 0.34335664 0.34405594 0.34475524 0.34545455 0.34615385 0.34685315 0.34755245 0.34825175 0.34895105 0.34965035 0.35034965 0.35104895 0.35174825 0.35244755 0.35314685 0.35384615 0.35454545 0.35524476 0.35594406 0.35664336 0.35734266 0.35804196 0.35874126 0.35944056 0.36013986 0.36083916 0.36153846 0.36223776 0.36293706 0.36363636 0.36433566 0.36503497 0.36573427 0.36643357 0.36713287 0.36783217 0.36853147 0.36923077 0.36993007 0.37062937 0.37132867 0.37202797 0.37272727 0.37342657 0.37412587 0.37482517 0.37552448 0.37622378 0.37692308 0.37762238 0.37832168 0.37902098 0.37972028 0.38041958 0.38111888 0.38181818 0.38251748 0.38321678 0.38391608 0.38461538 0.38531469 0.38601399 0.38671329 0.38741259 0.38811189 0.38881119 0.38951049 0.39020979 0.39090909 0.39160839 0.39230769 0.39300699 0.39370629 0.39440559 0.3951049 0.3958042 0.3965035 0.3972028 0.3979021 0.3986014 0.3993007 0.4 0.4006993 0.4013986 0.4020979 0.4027972 0.4034965 0.4041958 0.4048951 0.40559441 0.40629371 0.40699301 0.40769231 0.40839161 0.40909091 0.40979021 0.41048951 0.41118881 0.41188811 0.41258741 0.41328671 0.41398601 0.41468531 0.41538462 0.41608392 0.41678322 0.41748252 0.41818182 0.41888112 0.41958042 0.42027972 0.42097902 0.42167832 0.42237762 0.42307692 0.42377622 0.42447552 0.42517483 0.42587413 0.42657343 0.42727273 0.42797203 0.42867133 0.42937063 0.43006993 0.43076923 0.43146853 0.43216783 0.43286713 0.43356643 0.43426573 0.43496503 0.43566434 0.43636364 0.43706294 0.43776224 0.43846154 0.43916084 0.43986014 0.44055944 0.44125874 0.44195804 0.44265734 0.44335664 0.44405594 0.44475524 0.44545455 0.44615385 0.44685315 0.44755245 0.44825175 0.44895105 0.44965035 0.45034965 0.45104895 0.45174825 0.45244755 0.45314685 0.45384615 0.45454545 0.45524476 0.45594406 0.45664336 0.45734266 0.45804196 0.45874126 0.45944056 0.46013986 0.46083916 0.46153846 0.46223776 0.46293706 0.46363636 0.46433566 0.46503497 0.46573427 0.46643357 0.46713287 0.46783217 0.46853147 0.46923077 0.46993007 0.47062937 0.47132867 0.47202797 0.47272727 0.47342657 0.47412587 0.47482517 0.47552448 0.47622378 0.47692308 0.47762238 0.47832168 0.47902098 0.47972028 0.48041958 0.48111888 0.48181818 0.48251748 0.48321678 0.48391608 0.48461538 0.48531469 0.48601399 0.48671329 0.48741259 0.48811189 0.48881119 0.48951049 0.49020979 0.49090909 0.49160839 0.49230769 0.49300699 0.49370629 0.49440559 0.4951049 0.4958042 0.4965035 0.4972028 0.4979021 0.4986014 0.4993007 0.5 0.5006993 0.5013986 0.5020979 0.5027972 0.5034965 0.5041958 0.5048951 0.50559441 0.50629371 0.50699301 0.50769231 0.50839161 0.50909091 0.50979021 0.51048951 0.51118881 0.51188811 0.51258741 0.51328671 0.51398601 0.51468531 0.51538462 0.51608392 0.51678322 0.51748252 0.51818182 0.51888112 0.51958042 0.52027972 0.52097902 0.52167832 0.52237762 0.52307692 0.52377622 0.52447552 0.52517483 0.52587413 0.52657343 0.52727273 0.52797203 0.52867133 0.52937063 0.53006993 0.53076923 0.53146853 0.53216783 0.53286713 0.53356643 0.53426573 0.53496503 0.53566434 0.53636364 0.53706294 0.53776224 0.53846154 0.53916084 0.53986014 0.54055944 0.54125874 0.54195804 0.54265734 0.54335664 0.54405594 0.54475524 0.54545455 0.54615385 0.54685315 0.54755245 0.54825175 0.54895105 0.54965035 0.55034965 0.55104895 0.55174825 0.55244755 0.55314685 0.55384615 0.55454545 0.55524476 0.55594406 0.55664336 0.55734266 0.55804196 0.55874126 0.55944056 0.56013986 0.56083916 0.56153846 0.56223776 0.56293706 0.56363636 0.56433566 0.56503497 0.56573427 0.56643357 0.56713287 0.56783217 0.56853147 0.56923077 0.56993007 0.57062937 0.57132867 0.57202797 0.57272727 0.57342657 0.57412587 0.57482517 0.57552448 0.57622378 0.57692308 0.57762238 0.57832168 0.57902098 0.57972028 0.58041958 0.58111888 0.58181818 0.58251748 0.58321678 0.58391608 0.58461538 0.58531469 0.58601399 0.58671329 0.58741259 0.58811189 0.58881119 0.58951049 0.59020979 0.59090909 0.59160839 0.59230769 0.59300699 0.59370629 0.59440559 0.5951049 0.5958042 0.5965035 0.5972028 0.5979021 0.5986014 0.5993007 0.6 0.6006993 0.6013986 0.6020979 0.6027972 0.6034965 0.6041958 0.6048951 0.60559441 0.60629371 0.60699301 0.60769231 0.60839161 0.60909091 0.60979021 0.61048951 0.61118881 0.61188811 0.61258741 0.61328671 0.61398601 0.61468531 0.61538462 0.61608392 0.61678322 0.61748252 0.61818182 0.61888112 0.61958042 0.62027972 0.62097902 0.62167832 0.62237762 0.62307692 0.62377622 0.62447552 0.62517483 0.62587413 0.62657343 0.62727273 0.62797203 0.62867133 0.62937063 0.63006993 0.63076923 0.63146853 0.63216783 0.63286713 0.63356643 0.63426573 0.63496503 0.63566434 0.63636364 0.63706294 0.63776224 0.63846154 0.63916084 0.63986014 0.64055944 0.64125874 0.64195804 0.64265734 0.64335664 0.64405594 0.64475524 0.64545455 0.64615385 0.64685315 0.64755245 0.64825175 0.64895105 0.64965035 0.65034965 0.65104895 0.65174825 0.65244755 0.65314685 0.65384615 0.65454545 0.65524476 0.65594406 0.65664336 0.65734266 0.65804196 0.65874126 0.65944056 0.66013986 0.66083916 0.66153846 0.66223776 0.66293706 0.66363636 0.66433566 0.66503497 0.66573427 0.66643357 0.66713287 0.66783217 0.66853147 0.66923077 0.66993007 0.67062937 0.67132867 0.67202797 0.67272727 0.67342657 0.67412587 0.67482517 0.67552448 0.67622378 0.67692308 0.67762238 0.67832168 0.67902098 0.67972028 0.68041958 0.68111888 0.68181818 0.68251748 0.68321678 0.68391608 0.68461538 0.68531469 0.68601399 0.68671329 0.68741259 0.68811189 0.68881119 0.68951049 0.69020979 0.69090909 0.69160839 0.69230769 0.69300699 0.69370629 0.69440559 0.6951049 0.6958042 0.6965035 0.6972028 0.6979021 0.6986014 0.6993007 0.7 0.7006993 0.7013986 0.7020979 0.7027972 0.7034965 0.7041958 0.7048951 0.70559441 0.70629371 0.70699301 0.70769231 0.70839161 0.70909091 0.70979021 0.71048951 0.71118881 0.71188811 0.71258741 0.71328671 0.71398601 0.71468531 0.71538462 0.71608392 0.71678322 0.71748252 0.71818182 0.71888112 0.71958042 0.72027972 0.72097902 0.72167832 0.72237762 0.72307692 0.72377622 0.72447552 0.72517483 0.72587413 0.72657343 0.72727273 0.72797203 0.72867133 0.72937063 0.73006993 0.73076923 0.73146853 0.73216783 0.73286713 0.73356643 0.73426573 0.73496503 0.73566434 0.73636364 0.73706294 0.73776224 0.73846154 0.73916084 0.73986014 0.74055944 0.74125874 0.74195804 0.74265734 0.74335664 0.74405594 0.74475524 0.74545455 0.74615385 0.74685315 0.74755245 0.74825175 0.74895105 0.74965035 0.75034965 0.75104895 0.75174825 0.75244755 0.75314685 0.75384615 0.75454545 0.75524476 0.75594406 0.75664336 0.75734266 0.75804196 0.75874126 0.75944056 0.76013986 0.76083916 0.76153846 0.76223776 0.76293706 0.76363636 0.76433566 0.76503497 0.76573427 0.76643357 0.76713287 0.76783217 0.76853147 0.76923077 0.76993007 0.77062937 0.77132867 0.77202797 0.77272727 0.77342657 0.77412587 0.77482517 0.77552448 0.77622378 0.77692308 0.77762238 0.77832168 0.77902098 0.77972028 0.78041958 0.78111888 0.78181818 0.78251748 0.78321678 0.78391608 0.78461538 0.78531469 0.78601399 0.78671329 0.78741259 0.78811189 0.78881119 0.78951049 0.79020979 0.79090909 0.79160839 0.79230769 0.79300699 0.79370629 0.79440559 0.7951049 0.7958042 0.7965035 0.7972028 0.7979021 0.7986014 0.7993007 0.8 0.8006993 0.8013986 0.8020979 0.8027972 0.8034965 0.8041958 0.8048951 0.80559441 0.80629371 0.80699301 0.80769231 0.80839161 0.80909091 0.80979021 0.81048951 0.81118881 0.81188811 0.81258741 0.81328671 0.81398601 0.81468531 0.81538462 0.81608392 0.81678322 0.81748252 0.81818182 0.81888112 0.81958042 0.82027972 0.82097902 0.82167832 0.82237762 0.82307692 0.82377622 0.82447552 0.82517483 0.82587413 0.82657343 0.82727273 0.82797203 0.82867133 0.82937063 0.83006993 0.83076923 0.83146853 0.83216783 0.83286713 0.83356643 0.83426573 0.83496503 0.83566434 0.83636364 0.83706294 0.83776224 0.83846154 0.83916084 0.83986014 0.84055944 0.84125874 0.84195804 0.84265734 0.84335664 0.84405594 0.84475524 0.84545455 0.84615385 0.84685315 0.84755245 0.84825175 0.84895105 0.84965035 0.85034965 0.85104895 0.85174825 0.85244755 0.85314685 0.85384615 0.85454545 0.85524476 0.85594406 0.85664336 0.85734266 0.85804196 0.85874126 0.85944056 0.86013986 0.86083916 0.86153846 0.86223776 0.86293706 0.86363636 0.86433566 0.86503497 0.86573427 0.86643357 0.86713287 0.86783217 0.86853147 0.86923077 0.86993007 0.87062937 0.87132867 0.87202797 0.87272727 0.87342657 0.87412587 0.87482517 0.87552448 0.87622378 0.87692308 0.87762238 0.87832168 0.87902098 0.87972028 0.88041958 0.88111888 0.88181818 0.88251748 0.88321678 0.88391608 0.88461538 0.88531469 0.88601399 0.88671329 0.88741259 0.88811189 0.88881119 0.88951049 0.89020979 0.89090909 0.89160839 0.89230769 0.89300699 0.89370629 0.89440559 0.8951049 0.8958042 0.8965035 0.8972028 0.8979021 0.8986014 0.8993007 0.9 0.9006993 0.9013986 0.9020979 0.9027972 0.9034965 0.9041958 0.9048951 0.90559441 0.90629371 0.90699301 0.90769231 0.90839161 0.90909091 0.90979021 0.91048951 0.91118881 0.91188811 0.91258741 0.91328671 0.91398601 0.91468531 0.91538462 0.91608392 0.91678322 0.91748252 0.91818182 0.91888112 0.91958042 0.92027972 0.92097902 0.92167832 0.92237762 0.92307692 0.92377622 0.92447552 0.92517483 0.92587413 0.92657343 0.92727273 0.92797203 0.92867133 0.92937063 0.93006993 0.93076923 0.93146853 0.93216783 0.93286713 0.93356643 0.93426573 0.93496503 0.93566434 0.93636364 0.93706294 0.93776224 0.93846154 0.93916084 0.93986014 0.94055944 0.94125874 0.94195804 0.94265734 0.94335664 0.94405594 0.94475524 0.94545455 0.94615385 0.94685315 0.94755245 0.94825175 0.94895105 0.94965035 0.95034965 0.95104895 0.95174825 0.95244755 0.95314685 0.95384615 0.95454545 0.95524476 0.95594406 0.95664336 0.95734266 0.95804196 0.95874126 0.95944056 0.96013986 0.96083916 0.96153846 0.96223776 0.96293706 0.96363636 0.96433566 0.96503497 0.96573427 0.96643357 0.96713287 0.96783217 0.96853147 0.96923077 0.96993007 0.97062937 0.97132867 0.97202797 0.97272727 0.97342657 0.97412587 0.97482517 0.97552448 0.97622378 0.97692308 0.97762238 0.97832168 0.97902098 0.97972028 0.98041958 0.98111888 0.98181818 0.98251748 0.98321678 0.98391608 0.98461538 0.98531469 0.98601399 0.98671329 0.98741259 0.98811189 0.98881119 0.98951049 0.99020979 0.99090909 0.99160839 0.99230769 0.99300699 0.99370629 0.99440559 0.9951049 0.9958042 0.9965035 0.9972028 0.9979021 0.9986014 0.9993007 1 1 1 1 1 1